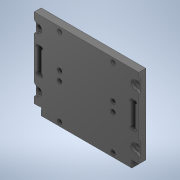
# Autodesk Inventor part: Cockpit_horizontal_frame_05
Saved by Autodesk Inventor 2020.4 (Build 244396000, 396)
## iProperties
Created: 2021-08-14
Part Number: Cockpit_horizontal_frame_05
Material: アセタール樹脂、黒
Document SubType Name: Modeling
Designer: Masato Kubotera
Density: 1.425 g/cm^3
Appearance: 滑らか - 黒
Mass: 37.8231 g
Surface Area: 126.929 cm^2
Volume: 26.5425 cm^3
Description: POM T5
Author: Masato Kubotera
Title: Cockpit_horizontal_frame_05
Autodesk Inventor part; units mm, degrees
ref_plane "YZ Plane" through (0, 0, 0) normal (1, 0, 0) x (0, 1, 0)
ref_plane "XZ Plane" through (0, 0, 0) normal (0, 1, 0) x (-1, 0, 0)
ref_plane "XY Plane" through (0, 0, 0) normal (0, 0, 1) x (1, 0, 0)
sketch "スケッチ1" plane through (0, 0, 0) normal (0, 0, 1) x (1, 0, 0)
  line L0 (37.25, 28.25) -> (37.25, 23.75)
  line L1 (-37.25, -28.25) -> (-37.25, -11.5167)
  line L2 (-37.25, 28.25) -> (37.25, -28.25) construction
  line L3 (37.25, 28.25) -> (-37.25, -28.25) construction
  line L4 (0, 28.25) -> (0, -28.25) construction
  line L5 (-37.25, 11.5167) -> (-37.25, 28.25)
  line L6 (-37.25, -11.5167) -> (-37.25, 11.5167)
  line L7 (37.25, 11.5167) -> (37.25, -11.5167)
  line L8 (37.25, -11.5167) -> (37.25, -28.25)
  line L9 (-37.25, 0) -> (37.25, 0) construction
  line L10 (37.25, 23.75) -> (37.25, 11.5167)
  line L11 (-24.5, -2.25) -> (24.5, -2.25) construction
  line L12 (24.5, -2.25) -> (24.5, -33.25) construction
  line L13 (24.5, -33.25) -> (-24.5, -33.25) construction
  line L14 (-24.5, -33.25) -> (-24.5, -2.25) construction
  line L15 (-24.5, -2.25) -> (24.5, -33.25) construction
  line L16 (24.5, -2.25) -> (-24.5, -33.25) construction
  circle A0 centre (-19, -5.25) radius 1.55
  line L17 (24.5, -17.75) -> (-24.5, -17.75) construction
  circle A1 centre (-19, -30.25) radius 1.55
  circle A2 centre (19, -5.25) radius 1.55
  circle A3 centre (19, -30.25) radius 1.55
  line L18 (-34.75, 9.4167) -> (-32.25, 9.4167) construction
  line L19 (-32.25, 9.4167) -> (-32.25, -9.4167) construction
  line L20 (-32.25, -9.4167) -> (-34.75, -9.4167) construction
  line L21 (-34.75, -9.4167) -> (-34.75, 9.4167) construction
  line L22 (-34.75, 9.4167) -> (-32.25, -9.4167) construction
  line L23 (-32.25, 9.4167) -> (-34.75, -9.4167) construction
  line L24 (-34.76, 9.4267) -> (-32.24, 9.4267)
  line L25 (-32.24, 9.4267) -> (-32.24, 7.3267) construction
  line L26 (-32.24, -9.4267) -> (-34.76, -9.4267)
  line L27 (-34.76, -9.4267) -> (-34.76, -7.3267) construction
  line L28 (-34.76, 9.4267) -> (-32.24, -9.4267) construction
  line L29 (-32.24, 9.4267) -> (-34.76, -9.4267) construction
  arc A4 (-34.76, 9.4267) -> (-34.76, 7.3267) centre (-34.76, 8.3767) ccw
  line L30 (-33.5, 9.4167) -> (-33.5, -9.4167) construction
  line L31 (-34.75, 0) -> (-32.25, 0) construction
  arc A5 (-32.24, 7.3267) -> (-32.24, 9.4267) centre (-32.24, 8.3767) ccw
  arc A6 (-34.76, -7.3267) -> (-34.76, -9.4267) centre (-34.76, -8.3767) ccw
  arc A7 (-32.24, -9.4267) -> (-32.24, -7.3267) centre (-32.24, -8.3767) ccw
  line L32 (-34.76, 7.3267) -> (-34.76, 9.4267) construction
  line L33 (-32.24, 7.3267) -> (-32.24, -7.3267)
  line L34 (-34.76, -7.3267) -> (-34.76, 7.3267)
  line L35 (-32.24, -7.3267) -> (-32.24, -9.4267) construction
  line L36 (34.75, 9.4167) -> (32.25, 9.4167) construction
  line L37 (32.25, 9.4167) -> (32.25, -9.4167) construction
  line L38 (32.25, -9.4167) -> (34.75, -9.4167) construction
  line L39 (34.75, -9.4167) -> (34.75, 9.4167) construction
  line L40 (34.75, 9.4167) -> (32.25, -9.4167) construction
  line L41 (32.25, 9.4167) -> (34.75, -9.4167) construction
  line L42 (34.76, 9.4267) -> (32.24, 9.4267)
  line L43 (32.24, 9.4267) -> (32.24, 7.3267) construction
  line L44 (32.24, -9.4267) -> (34.76, -9.4267)
  line L45 (34.76, -9.4267) -> (34.76, -7.3267) construction
  line L46 (34.76, 9.4267) -> (32.24, -9.4267) construction
  line L47 (32.24, 9.4267) -> (34.76, -9.4267) construction
  arc A8 (34.76, 7.3267) -> (34.76, 9.4267) centre (34.76, 8.3767) ccw
  line L48 (33.5, 9.4167) -> (33.5, -9.4167) construction
  line L49 (34.75, 0) -> (32.25, 0) construction
  arc A9 (32.24, 9.4267) -> (32.24, 7.3267) centre (32.24, 8.3767) ccw
  arc A10 (34.76, -9.4267) -> (34.76, -7.3267) centre (34.76, -8.3767) ccw
  arc A11 (32.24, -7.3267) -> (32.24, -9.4267) centre (32.24, -8.3767) ccw
  line L50 (34.76, 7.3267) -> (34.76, 9.4267) construction
  line L51 (32.24, 7.3267) -> (32.24, -7.3267)
  line L52 (34.76, -7.3267) -> (34.76, 7.3267)
  line L53 (32.24, -7.3267) -> (32.24, -9.4267) construction
  circle A12 centre (-34.75, 19.4167) radius 1.55
  circle A13 centre (-34.75, 19.4167) radius 3
  circle A14 centre (34.75, 19.4167) radius 1.55
  circle A15 centre (34.75, 19.4167) radius 3
  circle A16 centre (-34.75, -19.4167) radius 3
  circle A17 centre (34.75, -19.4167) radius 3
  circle A18 centre (34.75, -19.4167) radius 1.55
  circle A19 centre (-34.75, -19.4167) radius 1.55
  line L54 (37.25, 28.25) -> (-37.25, 28.25)
  line L55 (-32.25, -29.7349) -> (-32.25, -33.25)
  line L56 (-32.25, -33.25) -> (32.25, -33.25)
  line L57 (-37.25, -28.25) -> (-33.7349, -28.25)
  arc A20 (-32.25, -29.7349) -> (-33.7349, -28.25) centre (-32.9925, -28.9925) ccw
  line L58 (32.25, -29.7349) -> (32.25, -33.25)
  line L59 (37.25, -28.25) -> (33.7349, -28.25)
  arc A21 (33.7349, -28.25) -> (32.25, -29.7349) centre (32.9925, -28.9925) ccw
  line L60 (-24.5, 28.25) -> (24.5, 28.25) construction
  line L61 (24.5, 28.25) -> (24.5, -1.75) construction
  line L62 (24.5, -1.75) -> (-24.5, -1.75) construction
  line L63 (-24.5, -1.75) -> (-24.5, 28.25) construction
  line L64 (-24.5, 28.25) -> (24.5, -1.75) construction
  line L65 (24.5, 28.25) -> (-24.5, -1.75) construction
  circle A22 centre (-19, 25.25) radius 1.55
  line L66 (-24.5, 13.25) -> (24.5, 13.25) construction
  circle A23 centre (-19, 1.25) radius 1.55
  circle A24 centre (19, 25.25) radius 1.55
  circle A25 centre (19, 1.25) radius 1.55
  point P0 (0, 0)
  point P1 (0, 0)
  point P2 (0, 0)
  point P3 (0, 0)
  point P4 (0, -17.75)
  point P5 (-33.5, 0)
  point P6 (-33.5, 0)
  point P7 (-33.5, 0)
  point P8 (33.5, 0)
  point P9 (33.5, 0)
  point P10 (33.5, 0)
  point P11 (-33.5, 0)
  point P12 (37.25, 17.7584)
  point P13 (37.25, 21.075)
  point P14 (37.25, -21.075)
  point P15 (37.25, -17.7584)
  point P16 (-37.25, -17.7584)
  point P17 (-37.25, -21.075)
  point P18 (-37.25, 21.075)
  point P19 (-37.25, 17.7584)
  point P20 (-37.25, 21.075)
  point P21 (-32.25, -28.25)
  point P22 (0, 13.25)
  dimension "d96" = 6
  dimension "d69" = 49
  dimension "d70" = 31
  dimension "d73" = 3.1
  dimension "d82" = 2.5
  dimension "d83" = 18.8333
  dimension "d84" = 1.05
  dimension "d87" = 0.01
  dimension "d88" = 0.01
  dimension "d89" = 64.5
  dimension "d95" = 3.1
  dimension "d97" = 10
  dimension "d102" = 2.5
  dimension "d103" = 5
  dimension "d109" = 56.5
  dimension "d110" = 38
  dimension "d111" = 25
  dimension "d113" = 0
  dimension "d114" = 1.05
  dimension "d115" = 5
  dimension "d116" = 30
  dimension "d117" = 0.5
  dimension "d118" = 3.1
  dimension "d119" = 38
  dimension "d120" = 24
  constraints: 134 end point, 48 symmetric about line, 35 midpoint, 28 parallel, 25 centre point, 21 point on circle, 8 perpendicular, 8 point on line, 6 horizontal, 3 coincident, 2 collinear, 1 vertical, 23 other
  measures "d69" distance of L12.end L13.end
  measures "d70" distance of L11.end L12.end
  measures "d73" diameter of A0
  measures "d82" distance of L19.end L20.end
  measures "d83" distance of L18.end L19.end
  measures "d84" radius of A4
  measures "d87" distance between parallel lines of L18 L24
  measures "d88" distance between parallel lines of L21 L34
  measures "d89" distance between parallel lines of L19 L37
  measures "d95" diameter of A12
  measures "d97" distance from line of A12.centre L18
  measures "d102" distance from line of L19 A12.centre
  measures "d103" distance from line of L19 L2.start
  measures "d109" distance of L2.end L0.start
  measures "d110" distance of A2.centre A0.centre
  measures "d111" distance of A3.centre A2.centre
  measures "d113" distance between parallel lines of L56 L13
  measures "d114" radius of A20
  measures "d115" distance from line of L1.start L56
  measures "d116" distance of L60.end L61.end
  measures "d117" distance between parallel lines of L11 L62
  measures "d118" diameter of A22
  measures "d119" distance of A24.centre A22.centre
  measures "d120" distance of A23.centre A22.centre
extrude "押し出し1" add sketch "スケッチ1" along normal blind 5 contours L0 L10 A15 L7 L8 A17 L59 A21 L58 L56 L55 A20 L57 L1 A16 L6 L5 A13 L54
extrude "押し出し3" add sketch "スケッチ1" along normal blind 3.5 contours L10 A15 | A13 L5 | L8 A17 | A16 L1 picked at (36.9333, 19.4167) picked at (-36.9333, 19.4167) picked at (36.9333, -19.4167) picked at (-36.9333, -19.4167)
fillet "フィレット5" radius 2 8 edges at (-37.25, -17.7584, 4.25) (-37.25, -21.075, 4.25) (37.25, -21.075, 4.25) (37.25, -17.7584, 4.25) (-37.25, 21.075, 4.25) (-37.25, 17.7584, 4.25) (37.25, 17.7584, 4.25) (37.25, 21.075, 4.25)
